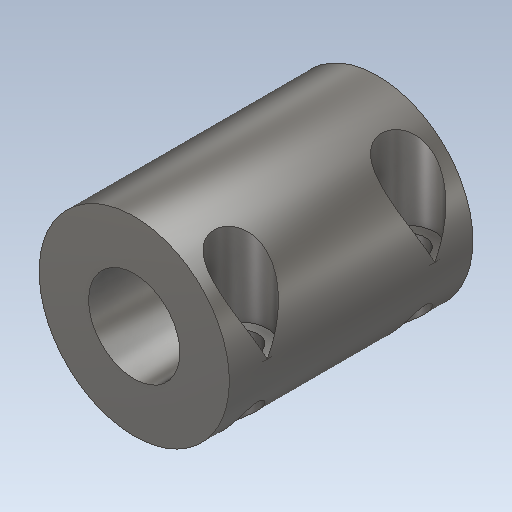
# Autodesk Inventor part: Cartesian1_12_12_Clutch
Saved by Autodesk Inventor 2020 (Build 240168000, 168)
## iProperties
Created: 2020-02-29
Part Number: Cartesian1_12_12_Clutch
Material: Stal, stopowa
Document SubType Name: Modeling
Designer: invin
Density: 7.73 g/cm^3
Appearance: Częściowo polerowana
Mass: 86.4846 g
Surface Area: 48.8026 cm^2
Volume: 11.1882 cm^3
Author: invin
Autodesk Inventor part; units mm, degrees
ref_plane "YZ Plane" through (0, 0, 0) normal (1, 0, 0) x (0, 1, 0)
ref_plane "XZ Plane" through (0, 0, 0) normal (0, 1, 0) x (-1, 0, 0)
ref_plane "XY Plane" through (0, 0, 0) normal (0, 0, 1) x (1, 0, 0)
sketch "Szkic1" plane through (0, 0, 0) normal (0, 0, 1) x (1, 0, 0)
  circle A0 centre (0, 0) radius 12.5
  dimension "d0" = 25
  constraints: 1 centre point, 1 coincident
  measures "d0" diameter of A0
extrude "Wyciągnięcie proste1" add sketch "Szkic1" along normal blind 32
sketch "Szkic2" plane through (0, 0, 32) normal (0, 0, 1) x (1, 0, 0)
  circle A0 centre (0, 0) radius 6
  dimension "d3" = 12
  constraints: 1 centre point, 1 coincident
  measures "d3" diameter of A0
extrude "Wyciągnięcie proste2" cut sketch "Szkic2" against normal blind 32
sketch "Szkic3" plane through (0, 0, 0) normal (0, 1, 0) x (-1, 0, 0)
  circle A0 centre (-9, 5) radius 2
  circle A1 centre (-9, 27) radius 2
  line L0 (0, 0) -> (0, -10.8071)
  circle A2 centre (-9, 27) radius 3.5
  circle A3 centre (-9, 5) radius 3.5
  line L1 (-12.5, 0) -> (12.5, 0) projected
  line L2 (12.5, 32) -> (-12.5, 32) projected
  dimension "d6" = 4
  dimension "d7" = 4
  dimension "d8" = 9
  dimension "d9" = 9
  dimension "d10" = 7
  dimension "d11" = 7
  dimension "d12" = 5
  dimension "d13" = 5
  constraints: 4 centre point, 2 concentric, 2 end point, 1 vertical
  measures "d6" diameter of A0
  measures "d7" diameter of A1
  measures "d8" distance from line of L0 A0.centre
  measures "d9" distance from line of L0 A1.centre
  measures "d10" diameter of A2
  measures "d11" diameter of A3
  measures "d12" distance from line of L1 A3.centre
  measures "d13" distance from line of L2 A2.centre
extrude "Wyciągnięcie proste3" cut sketch "Szkic3" along normal blind 32 contours A0 | A1 | A2 | A3
sketch "Szkic4" plane through (0, 0, 0) normal (0, 1, 0) x (1, 0, 0)
  circle A0 centre (9, -27) radius 2.25
  circle A1 centre (9, -5) radius 2.25
  arc A2 (6, -6.8028) -> (12.5, -5) centre (9, -5) ccw projected
  arc A3 (12.5, -27) -> (6, -25.1972) centre (9, -27) ccw projected
  point P0 (0, 0)
  dimension "d16" = 4.5
  dimension "d17" = 4.5
  constraints: 2 centre point, 2 concentric
  measures "d16" diameter of A0
  measures "d17" diameter of A1
extrude "Wyciągnięcie proste4" cut sketch "Szkic4" against normal blind 32
